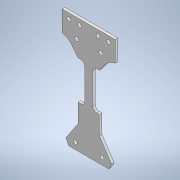
# Autodesk Inventor part: body_bone_4
Saved by Autodesk Inventor 2020 (Build 240168000, 168)
## iProperties
Created: 2019-05-16
Part Number: body_bone_4
Material: Generic
Document SubType Name: Modeling
Designer: psrob
Density: 1 g/cm^3
Appearance: Default
Author: psrob
Autodesk Inventor part; units mm, degrees
ref_plane "YZ Plane" through (0, 0, 0) normal (1, 0, 0) x (0, 1, 0)
ref_plane "XZ Plane" through (0, 0, 0) normal (0, 1, 0) x (-1, 0, 0)
ref_plane "XY Plane" through (0, 0, 0) normal (0, 0, 1) x (1, 0, 0)
sketch "Sketch1" plane through (0, 0, 0) normal (0, 0, 1) x (1, 0, 0)
  circle A0 centre (-14, 4) radius 1.5 projected
  circle A1 centre (-10, 13) radius 1.5 projected
  circle A2 centre (-7, 4) radius 1.5 projected
  line L0 (-20, 0) -> (-20, 8) projected
  line L1 (0, 0) -> (-20, 0) projected
  line L2 (0, 40) -> (0, 0) projected
  line L3 (-10, 40) -> (0, 40) projected
  line L4 (-10, 23) -> (-10, 40) projected
  line L5 (-10, 23) -> (-20, 8) projected
  circle A3 centre (14, 4) radius 1.5 projected
  circle A4 centre (10, 13) radius 1.5 projected
  circle A5 centre (7, 4) radius 1.5 projected
  line L6 (20, 0) -> (20, 8) projected
  line L7 (10, 23) -> (20, 8) projected
  line L8 (10, 23) -> (10, 40) projected
  line L9 (10, 40) -> (0, 40) projected
  line L10 (0, 40) -> (0, 0) projected
  line L11 (0, 0) -> (20, 0) projected
  line L12 (3, 84.8834) -> (-3, 84.8834) projected
  line L13 (-3, 84.8834) -> (-3, -165.1166) projected
  line L14 (3, -165.1166) -> (-3, -165.1166) projected
  line L15 (3, 84.8834) -> (3, -165.1166) projected
  circle A6 centre (-9, 80.8834) radius 1.5 projected
  circle A7 centre (-7, 90.8834) radius 1.5 projected
  circle A8 centre (-15, 90.8834) radius 1.5 projected
  line L16 (-12.05, 74.2834) -> (-8.0217, 68.9123) projected
  line L17 (-8.0217, 68.9123) -> (0, 68.9123) projected
  line L18 (0, 94.8834) -> (0, 68.9123) projected
  line L19 (0, 94.8834) -> (-20, 94.8834) projected
  line L20 (-20, 79.501) -> (-20, 94.8834) projected
  arc A9 (-12.05, 74.2834) -> (-20, 79.501) centre (-23.25, 65.8834) ccw projected
  line L21 (3, 94.8834) -> (3, 68.9123) projected
  circle A10 centre (9, 80.8834) radius 1.5 projected
  circle A11 centre (7, 90.8834) radius 1.5 projected
  circle A12 centre (15, 90.8834) radius 1.5 projected
  line L22 (12.05, 74.2834) -> (8.0217, 68.9123) projected
  arc A13 (20, 79.501) -> (12.05, 74.2834) centre (23.25, 65.8834) ccw projected
  line L23 (20, 79.501) -> (20, 94.8834) projected
  line L24 (0, 94.8834) -> (20, 94.8834) projected
  line L25 (0, 94.8834) -> (0, 68.9123) projected
  line L26 (8.0217, 68.9123) -> (0, 68.9123) projected
  line L27 (-20, 8) -> (20, 8)
  line L28 (-3, 40) -> (3, 40)
  line L29 (3, 40) -> (3, 68.9123)
  line L30 (3, 68.9123) -> (-3, 68.9123)
  line L31 (-3, 68.9123) -> (-3, 40)
  point P0 (3, 40)
  point P1 (-3, 68.9123)
  constraints: 10 end point, 2 parallel, 2 perpendicular, 2 point on line, 1 horizontal
extrude "Extrusion1" add sketch "Sketch1" along normal blind 2 contours L5 L4 L3 L13 L27 | L13 L3 L2 L27 | L13 L17 L26 L15 L9 L3 | L2 L9 L15 L27 | L17 L16 A9 L20 L19 L18 L12 L13 | L13 L12 L18 L17 | L15 L9 L8 L7 L27 | L18 L12 L15 L26 | L15 L21 L24 L23 A13 L22 L26 | L18 L24 L21 L12
chamfer "Chamfer1" distance 5 angle 45 2 edges at (20, 8, 1) (-20, 8, 1)
fillet "Fillet1" radius 3 4 edges at (3, 40, 1) (-3, 40, 1) (-3, 68.9123, 1) (3, 68.9123, 1)
body "Solid1"
